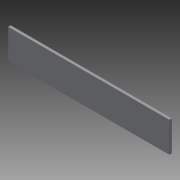
# Autodesk Inventor part: FE-00036Base
Saved by Autodesk Inventor 2013 (Build 170138000, 138)
## iProperties
Created: 2013-01-13
Part Number: FE-00036Base
Material: Generic
Document SubType Name: Modeling
Designer: Phillip
Density: 1 g/cm^3
d0: 16.000 in
d1: 3.000 in
d2: 1.000 in
d3: 0.250 in
d4: 0.00 deg
Author: Phillip
Autodesk Inventor part; units mm, degrees
ref_plane "YZ Plane" through (0, 0, 0) normal (1, 0, 0) x (0, 1, 0)
ref_plane "XZ Plane" through (0, 0, 0) normal (0, 1, 0) x (-1, 0, 0)
ref_plane "XY Plane" through (0, 0, 0) normal (0, 0, 1) x (1, 0, 0)
sketch "Sketch1" plane through (0, 0, 0) normal (0, 0, 1) x (1, 0, 0)
  line L0 (47.625, 38.1) -> (454.025, 38.1)
  line L1 (454.025, 38.1) -> (454.025, -38.1)
  line L2 (454.025, -38.1) -> (47.625, -38.1)
  line L3 (47.625, -38.1) -> (47.625, 38.1)
  line L4 (22.225, -22.225) -> (22.225, 22.225) projected
  point P0 (0, 0)
  point P1 (47.625, 0)
  dimension "d0" = 406.4
  dimension "d1" = 76.2
  dimension "d2" = 25.4
  constraints: 8 end point, 2 parallel, 1 horizontal, 1 horizontal alignment, 1 midpoint, 1 perpendicular
  measures "d0" distance of L1.end L2.end
  measures "d1" distance of L0.end L1.end
  measures "d2" distance between parallel lines of L3 L4
extrude "Extrusion1" add sketch "Sketch1" against normal blind 6.35
body "Solid1"
